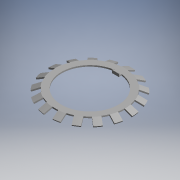
# Autodesk Inventor part: Washer50w
Saved by Autodesk Inventor 2017.3 (Build 213256000, 256)
## iProperties
Part Number: Washer50w
Material: Generic
Catalog Web Link: www.cadenas.de
Description: JLNK, JLNSK_washer-Tooth Lock Washers for Bearings
Vendor: MISUMI
Document SubType Name: Modeling
Designer: partserver
Manufacturer: MISUMI
Mass: 2.01723 g
Surface Area: 40.7557 cm^2
Volume: 2.01723 cm^3
Density: 1 g/cm^3
Appearance: PSOLRGB-192-192-192
Category: PARTsolutions
Company: MISUMI
Title: Washer50w
Author: Cadenas PARTsolutions
Comments: Tooth Lock Washers for Bearings
PSOL_IDENT_0: {$CADENAS_DATA\23d-libs\misumi\metric\12_bearing_holders\jlnk_w.prj},171 {VTYP=3D},{NB=Washer50w},{L
PSOL_IDENT_1: INA=Washer50w},{NN=JLNK, JLNSK_washer},{DATE=25.04.2017 02:57:38},{GEOMDATE=21.10.2008 15:30:00},{VE
PSOL_IDENT_2: RSION=},{LINEID=110},{WBVAR=},{WBNUMERIC=}  {NB=Washer50w},{LINA=Washer50w},{KT=DUMMY},{PN=Washer50}
PSOL_IDENT_3: ,{NO=50},{DD1=50},{KK=47.5},{S1=6},{S2=6},{TT=1.2},{V=2.5},{D3=74},{D4=61},{NOTH=17},{BB=2.0}
NB: Washer50w
NN: JLNK, JLNSK_washer
NT: Tooth Lock Washers for Bearings
NBSYN: $PN.w
LINA: Washer50w
CATALOG: Misumi
NO: 50
DD1: 50
KK: 47.5
S1: 6
S2: 6
TT: 1.2
V: 2.5
D3: 74
D4: 61
NOTH: 17
BB: 2
SUPPLIER: MISUMI
ARTICLENO: Washer50w
BOMINFO: Washer50w
CREATOR: CADENAS GmbH
Autodesk Inventor part; units mm, degrees
sketch "Sketch_1" plane through (0, 0, 0) normal (1, 0, 0) x (0, 1, 0)
  line L0 (0, 0) -> (0, 10)
  line L1 (36.4929, 3.9945) -> (30.5, 1.2)
  line L2 (30.5, 1.2) -> (25, 1.2)
  line L3 (25, 1.2) -> (25, 0)
  line L4 (25, 0) -> (30.766, 0)
  line L5 (30.766, 0) -> (37, 2.9069)
  line L6 (37, 2.9069) -> (36.4929, 3.9945)
  constraints: 14 end point
revolve "Revolution1" add sketch "Sketch_1" angle 360 about axis through (0, 0, 0) along (0, 0, -1)
sketch "Sketch_2" plane through (0, 0, 0) normal (1, 0, 0) x (0, 1, 0)
  line L0 (25, 1.2) -> (22.5, 1.2)
  line L1 (22.5, 1.2) -> (22.5, -1.3)
  line L2 (22.5, -1.3) -> (23.25, -1.3)
  line L3 (23.25, -1.3) -> (23.25, 0)
  line L4 (23.25, 0) -> (25, 0)
  line L5 (25, 0) -> (25, 1.2)
  constraints: 12 end point
extrude "Extrusion1" add sketch "Sketch_2" along normal mid plane 6
sketch "Sketch_3" plane through (0, 0, 0) normal (0, 0, 1) x (1, 0, 0)
  circle A0 centre (0, 0) radius 74
  line L0 (-36.9977, 0.4155) -> (-30.4994, -0.1867)
  arc A1 (-30.4994, -0.1867) -> (-30.0144, -5.4208) centre (0, 0) ccw
  line L1 (-30.0144, -5.4208) -> (-36.2914, -7.2067)
  arc A2 (-36.2914, -7.2067) -> (-34.6494, -12.9777) centre (0, 0) ccw
  line L2 (-34.6494, -12.9777) -> (-28.3724, -11.1917)
  arc A3 (-28.3724, -11.1917) -> (-26.0294, -15.8972) centre (0, 0) ccw
  line L3 (-26.0294, -15.8972) -> (-31.2373, -19.83)
  arc A4 (-31.2373, -19.83) -> (-27.6215, -24.6181) centre (0, 0) ccw
  line L4 (-27.6215, -24.6181) -> (-22.4136, -20.6853)
  arc A5 (-22.4136, -20.6853) -> (-18.529, -24.2266) centre (0, 0) ccw
  line L5 (-18.529, -24.2266) -> (-21.9645, -29.7752)
  arc A6 (-21.9645, -29.7752) -> (-16.8632, -32.9338) centre (0, 0) ccw
  line L6 (-16.8632, -32.9338) -> (-13.4277, -27.3852)
  arc A7 (-13.4277, -27.3852) -> (-8.5261, -29.284) centre (0, 0) ccw
  line L7 (-8.5261, -29.284) -> (-9.7253, -35.699)
  arc A8 (-9.7253, -35.699) -> (-3.8274, -36.8015) centre (0, 0) ccw
  line L8 (-3.8274, -36.8015) -> (-2.6283, -30.3865)
  arc A9 (-2.6283, -30.3865) -> (2.6283, -30.3865) centre (0, 0) ccw
  line L9 (2.6283, -30.3865) -> (3.8274, -36.8015)
  arc A10 (3.8274, -36.8015) -> (9.7253, -35.699) centre (0, 0) ccw
  line L10 (9.7253, -35.699) -> (8.5261, -29.284)
  arc A11 (8.5261, -29.284) -> (13.4277, -27.3852) centre (0, 0) ccw
  line L11 (13.4277, -27.3852) -> (16.8632, -32.9338)
  arc A12 (16.8632, -32.9338) -> (21.9645, -29.7752) centre (0, 0) ccw
  line L12 (21.9645, -29.7752) -> (18.529, -24.2266)
  arc A13 (18.529, -24.2266) -> (22.4136, -20.6853) centre (0, 0) ccw
  line L13 (22.4136, -20.6853) -> (27.6215, -24.6181)
  arc A14 (27.6215, -24.6181) -> (31.2373, -19.83) centre (0, 0) ccw
  line L14 (31.2373, -19.83) -> (26.0294, -15.8972)
  arc A15 (26.0294, -15.8972) -> (28.3724, -11.1917) centre (0, 0) ccw
  line L15 (28.3724, -11.1917) -> (34.6494, -12.9777)
  arc A16 (34.6494, -12.9777) -> (36.2914, -7.2067) centre (0, 0) ccw
  line L16 (36.2914, -7.2067) -> (30.0144, -5.4208)
  arc A17 (30.0144, -5.4208) -> (30.4994, -0.1867) centre (0, 0) ccw
  line L17 (30.4994, -0.1867) -> (36.9977, 0.4155)
  arc A18 (36.9977, 0.4155) -> (36.4441, 6.3899) centre (0, 0) ccw
  line L18 (36.4441, 6.3899) -> (29.9458, 5.7877)
  arc A19 (29.9458, 5.7877) -> (28.5073, 10.8436) centre (0, 0) ccw
  line L19 (28.5073, 10.8436) -> (34.3492, 13.7525)
  arc A20 (34.3492, 13.7525) -> (31.6748, 19.1235) centre (0, 0) ccw
  line L20 (31.6748, 19.1235) -> (25.8329, 16.2146)
  arc A21 (25.8329, 16.2146) -> (22.6651, 20.4094) centre (0, 0) ccw
  line L21 (22.6651, 20.4094) -> (27.0617, 25.2322)
  arc A22 (27.0617, 25.2322) -> (22.6276, 29.2744) centre (0, 0) ccw
  line L22 (22.6276, 29.2744) -> (18.2311, 24.4516)
  arc A23 (18.2311, 24.4516) -> (13.7619, 27.2188) centre (0, 0) ccw
  line L23 (13.7619, 27.2188) -> (16.1194, 33.3042)
  arc A24 (16.1194, 33.3042) -> (10.5245, 35.4716) centre (0, 0) ccw
  line L24 (10.5245, 35.4716) -> (8.167, 29.3862)
  arc A25 (8.167, 29.3862) -> (3, 30.3521) centre (0, 0) ccw
  line L25 (3, 30.3521) -> (3, 36.8782)
  arc A26 (3, 36.8782) -> (-3, 36.8782) centre (0, 0) ccw
  line L26 (-3, 36.8782) -> (-3, 30.3521)
  arc A27 (-3, 30.3521) -> (-8.167, 29.3862) centre (0, 0) ccw
  line L27 (-8.167, 29.3862) -> (-10.5245, 35.4716)
  arc A28 (-10.5245, 35.4716) -> (-16.1194, 33.3042) centre (0, 0) ccw
  line L28 (-16.1194, 33.3042) -> (-13.7619, 27.2188)
  arc A29 (-13.7619, 27.2188) -> (-18.2311, 24.4516) centre (0, 0) ccw
  line L29 (-18.2311, 24.4516) -> (-22.6276, 29.2744)
  arc A30 (-22.6276, 29.2744) -> (-27.0617, 25.2322) centre (0, 0) ccw
  line L30 (-27.0617, 25.2322) -> (-22.6651, 20.4094)
  arc A31 (-22.6651, 20.4094) -> (-25.8329, 16.2146) centre (0, 0) ccw
  line L31 (-25.8329, 16.2146) -> (-31.6748, 19.1235)
  arc A32 (-31.6748, 19.1235) -> (-34.3492, 13.7525) centre (0, 0) ccw
  line L32 (-34.3492, 13.7525) -> (-28.5073, 10.8436)
  arc A33 (-28.5073, 10.8436) -> (-29.9458, 5.7877) centre (0, 0) ccw
  line L33 (-29.9458, 5.7877) -> (-36.4441, 6.3899)
  arc A34 (-36.4441, 6.3899) -> (-36.9977, 0.4155) centre (0, 0) ccw
  constraints: 68 end point, 68 point on circle, 35 centre point
extrude "Extrusion2" cut sketch "Sketch_3" along normal blind 20
ref_plane "washer_XY" through (0, 0, 1.2) normal (0, 0, 1) x (1, 0, 0)
ref_plane "washer_YZ" through (0, 0, 1.2) normal (1, 0, 0) x (0, 1, 0)
ref_plane "washer_ZX" through (0, 0, 1.2) normal (0, 1, 0) x (0, 0, 1)
body "Solid1"
